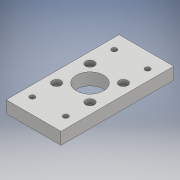
# Autodesk Inventor part: MOJ KOLNIERZ
Saved by Autodesk Inventor 2017 (Build 210142000, 142)
## iProperties
Created: 2018-05-29
Part Number: MOJ KOLNIERZ
Material: Generic
Document SubType Name: Modeling
Designer: Pies
Density: 1 g/cm^3
Appearance: Default
Author: Pies
Autodesk Inventor part; units mm, degrees
ref_plane "YZ Plane" through (0, 0, 0) normal (1, 0, 0) x (0, 1, 0)
ref_plane "XZ Plane" through (0, 0, 0) normal (0, 1, 0) x (-1, 0, 0)
ref_plane "XY Plane" through (0, 0, 0) normal (0, 0, 1) x (1, 0, 0)
sketch "Sketch1" plane through (0, 0, 0) normal (0, 0, 1) x (1, 0, 0)
  line L0 (0, -50) -> (-18, -50)
  line L1 (-18, -50) -> (-18, 50)
  line L2 (-18, 50) -> (18, 50)
  line L3 (18, 50) -> (18, -50)
  line L4 (18, -50) -> (0, -50)
  circle A0 centre (0, 0) radius 9
  constraints: 10 end point, 2 perpendicular, 1 centre point, 1 point on line
extrude "Extrusion2" add sketch "Sketch1" along normal blind 8
sketch "Sketch3" plane through (0, 0, 8) normal (0, 0, 1) x (1, 0, 0)
  line L0 (-18, 0) -> (18, 0) construction
  line L1 (18, 50) -> (18, -50) construction
  line L2 (-18, 50) -> (-18, -50) construction
  line L3 (-18, -50) -> (18, -50) projected
  line L4 (-18, -50) -> (18, -50)
  line L5 (18, -50) -> (18, -38)
  line L6 (18, -38) -> (-18, -38)
  line L7 (-18, -38) -> (-18, -50)
  line L8 (18, 50) -> (-18, 50) projected
  line L9 (-18, 50) -> (18, 50)
  line L10 (18, 50) -> (18, 38)
  line L11 (18, 38) -> (-18, 38)
  line L12 (-18, 38) -> (-18, 50)
  point P0 (0, 0)
  point P1 (-11, -27)
  point P2 (11.0001, -26.9664)
  point P3 (-11, 27)
  point P4 (11.0001, 26.9664)
  dimension "d57" = 36
  dimension "d58" = 12
  dimension "d59" = 36
  dimension "d60" = 12
  constraints: 18 end point, 4 parallel, 2 horizontal, 2 perpendicular, 1 midpoint
  measures "d57" distance of L6.end L5.end
  measures "d58" distance of L5.end L4.end
  measures "d59" distance of L10.end L11.end
  measures "d60" distance of L9.end L10.end
hole "Hole1" at (-11, -27, 8) at (11.0001, -26.9664, 8) at (-11, 27, 8) at (11.0001, 26.9664, 8) direction (0, 0, -1) diameter 3.4 end through all clearance for "Countersunk Flat Head Screw ISO 2009/7046" size "M3" standard "ISO"
sketch "Sketch6" plane through (0, 0, 0) normal (0, 0, -1) x (-1, 0, 0)
  circle A0 centre (-11, -11) radius 2.9
  circle A1 centre (11, -11) radius 2.9
  circle A2 centre (11, 11) radius 2.9
  circle A3 centre (-11, 11) radius 2.9
  point P0 (0, 0)
  constraints: 4 centre point
extrude "Extrusion5" cut sketch "Sketch6" against normal through all
sketch "Sketch7" plane through (0, 0, 0) normal (0, 0, -1) x (-1, 0, 0)
  circle A0 centre (-11, -11) radius 2.9 projected
  circle A1 centre (-11, -11) radius 5
  circle A2 centre (-11, 11) radius 2.9 projected
  circle A3 centre (-11, 11) radius 5
  circle A4 centre (11, 11) radius 2.9 projected
  circle A5 centre (11, 11) radius 5
  circle A6 centre (11, -11) radius 2.9 projected
  circle A7 centre (11, -11) radius 5
  point P0 (0, 0)
  dimension "d44" = 10
  dimension "d45" = 10
  dimension "d46" = 10
  dimension "d47" = 10
  constraints: 4 centre point, 4 coincident
  measures "d44" diameter of A1
  measures "d45" diameter of A3
  measures "d46" diameter of A5
  measures "d47" diameter of A7
extrude "Extrusion6" cut sketch "Sketch7" against normal blind 5
sketch "Sketch8" plane through (0, 0, 8) normal (0, 0, 1) x (1, 0, 0)
  line L0 (-18, 50) -> (-18, -50) projected
  line L1 (18, -49.142) -> (18, -37.142)
  line L2 (18, -37.142) -> (-18, -37.142)
  line L3 (-18, -37.142) -> (-18, -49.142)
  line L4 (18, 49.142) -> (18, 37.142)
  line L5 (18, 37.142) -> (-18, 37.142)
  line L6 (-18, 37.142) -> (-18, 49.142)
  line L7 (-18, -50) -> (18, -50) projected
  line L8 (18, -37.142) -> (-18, -37.142)
  line L9 (-18, -37.142) -> (-18, -50)
  line L10 (-18, -50) -> (18, -50)
  line L11 (18, -50) -> (18, -37.142)
  line L12 (-18, 50) -> (18, 50) projected
  line L13 (18, 37.142) -> (-18, 37.142)
  line L14 (-18, 37.142) -> (-18, 50)
  line L15 (-18, 50) -> (18, 50)
  line L16 (18, 50) -> (18, 37.142)
  point P0 (0, 0)
  dimension "d61" = 36
  dimension "d62" = 12
  dimension "d63" = 36
  dimension "d64" = 12
  constraints: 28 end point, 6 parallel, 2 horizontal, 2 perpendicular
  measures "d61" distance of L2.end L1.end
  measures "d62" distance of L1.end L1.start
  measures "d63" distance of L4.end L5.end
  measures "d64" distance of L4.start L4.end
extrude "Extrusion7" cut sketch "Sketch8" against normal through all
body "Solid2"
